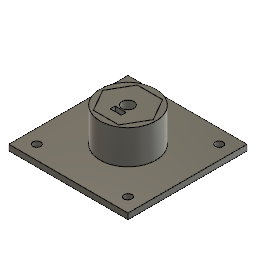
Rotation Motor Bottom Mount (Autodesk Fusion 360 design; units mm, degrees)
Autodesk Fusion 360 part; units mm, degrees
sketch "Sketch1" plane through (0, 0, 0) normal (0, 1, 0) x (1, 0, 0)
  circle A0 centre (-9.5106, -3.0902) radius 1.25
  circle A1 centre (0, 0) radius 14
  circle A2 centre (9.5106, -3.0902) radius 1.25
  circle A3 centre (5.8779, 8.0902) radius 1.25
  circle A4 centre (0, -10) radius 1.25
  circle A5 centre (5.8779, 8.0902) radius 1.25
  circle A6 centre (0, -10) radius 1.25
  circle A7 centre (-5.8779, 8.0902) radius 1.25
  circle A8 centre (9.5106, -3.0902) radius 1.25
  circle A9 centre (-9.5106, -3.0902) radius 1.25
  circle A10 centre (0, 0) radius 14
  circle A11 centre (-5.8779, 8.0902) radius 1.25
  circle A12 centre (-5.8779, 8.0902) radius 2.25
  circle A13 centre (5.8779, 8.0902) radius 2.25
  circle A14 centre (9.5106, -3.0902) radius 2.25
  circle A15 centre (0, -10) radius 2.25
  circle A16 centre (-9.5106, -3.0902) radius 2.25
  line L0 (30, -30) -> (-30, -30)
  line L1 (-30, -30) -> (-30, 30)
  line L2 (-30, 30) -> (30, 30)
  line L3 (30, 30) -> (30, -30)
  line L4 (30, -30) -> (-30, 30) construction
  line L5 (-30, -30) -> (30, 30) construction
  line L6 (-30, -30) -> (-22.9289, -22.9289)
  circle A17 centre (-22.9289, -22.9289) radius 1.95
  circle A18 centre (22.9289, -22.9289) radius 1.95
  circle A19 centre (22.9289, 22.9289) radius 1.95
  circle A20 centre (-22.9289, 22.9289) radius 1.95
  circle A21 centre (0, 0) radius 3
  line L7 (0, -3) -> (0, 2)
  line L8 (0, 2) -> (2.2361, 2)
  line L9 (0, 2) -> (-2.2361, 2)
  dimension "d13" = -1
  dimension "d14" = -1
  dimension "d15" = 1
  dimension "d16" = -1
  dimension "d17" = 1
  dimension "d33" = 60
  dimension "d34" = 60
  dimension "d35" = 10
  dimension "d36" = 3.9
  dimension "d50" = 6
  dimension "d51" = 5
  constraint horizontal L0
  constraint perpendicular L0 L1
  constraint parallel L0 L2
  constraint parallel L1 L3
  constraint parallel L5 L6
  constraint coincident L6.end A17.centre
  constraint coincident A1.centre A10.centre
  constraint coincident A21 L7.start
  constraint vertical L7
  constraint coincident A21 L8.end
  constraint perpendicular L7 L8
  constraint coincident A21 L9.end
  constraint perpendicular L7 L9
  measures "d33" distance of L1.end L2.end
  measures "d34" distance of L0.end L1.end
  measures "d35" distance of L0.end L6.end
  measures "d36" diameter of A17
  measures "d50" diameter of A21
  measures "d51" distance of L7.start L7.end
extrude "Extrude1" add sketch "Sketch1" along normal blind 17.065 contours A0 A9 | A1 A10 | A2 A8 | A3 A5 | A4 A6 | A7 A11 | A12 | A13 | A14 | A15 | A16 | A21 L7 L8 | A21 L8 L9 | A21 L7 L9 makes body 1
extrude "Extrude5" add sketch "Sketch1" 1 faces at (4.6394, 0, -2.5701) against normal blind 3 contours A0 A9 | A1 A10 | A2 A8 | A3 A5 | A4 A6 | A7 A11 | A12 | A13 | A14 | A15 | A16 | L0 L1 L2 L3 | A21 L7 L8 | A21 L8 L9 | A21 L7 L9 on bodies 1 bodies 1
sketch "Sketch3" plane through (0, 17.065, 0) normal (0, 1, 0) x (-1, 0, 0)
  circle A0 centre (0, 0) radius 14
  line L0 (6.3509, -11) -> (12.7017, 0)
  line L1 (12.7017, 0) -> (6.3509, 11)
  line L2 (6.3509, 11) -> (-6.3509, 11)
  line L3 (-6.3509, 11) -> (-12.7017, 0)
  line L4 (-12.7017, 0) -> (-6.3509, -11)
  line L5 (-6.3509, -11) -> (6.3509, -11)
  line L6 (-6.3797, 11.05) -> (-12.7594, 0)
  line L7 (-12.7594, 0) -> (-6.3797, -11.05)
  line L8 (-6.3797, -11.05) -> (6.3797, -11.05)
  line L9 (6.3797, -11.05) -> (12.7594, 0)
  line L10 (12.7594, 0) -> (6.3797, 11.05)
  line L11 (6.3797, 11.05) -> (-6.3797, 11.05)
  line L12 (0, -3) -> (0, 2)
  line L13 (0, 2) -> (2.2361, 2)
  circle A1 centre (0, 0) radius 3
  line L14 (0, 2) -> (-2.2361, 2)
  dimension "d55" = 11
  dimension "d56" = 0.05
  dimension "d61" = 6
  dimension "d62" = 5
  constraint coincident A0.centre A1.centre
  constraint coincident L12.start A1
  constraint vertical L12
  constraint coincident L13.end A1
  constraint perpendicular L12 L13
  constraint coincident L14.end A1
  constraint perpendicular L12 L14
  measures "d55" distance of A0.centre L5
  measures "d61" diameter of A1
  measures "d62" distance of L12.start L12.end
extrude "Extrude10" cut sketch "Sketch3" against normal blind 17.065 contours L0 L1 L2 L3 L4 L5 | L6 L7 L8 L9 L10 L11 | L12 A1 L14 | L12 L13 A1 | L13 A1 L14 bodies 1
extrude "Extrude11" add sketch "Sketch3" against normal blind 15 separate body contours L0 L1 L2 L3 L4 L5 | L12 A1 L14 | L12 L13 A1 | L13 A1 L14 makes body 2
extrude "Extrude12" cut sketch "Sketch3" against normal up to surface (15 mm away) contours L12 A1 L14 | L12 L13 A1 bodies 2
extrude "Extrude13" cut sketch "Sketch3" against normal blind 2 contours L13 A1 L14 bodies 2
sketch "Sketch4" plane through (0, 0, 11) normal (0, 0, 1) x (1, 0, 0)
  line L0 (6.3509, 17.065) -> (-6.3509, 17.065)
  line L1 (-6.3509, 17.065) -> (-6.3509, 2.065)
  line L2 (-6.3509, 2.065) -> (6.3509, 2.065)
  line L3 (6.3509, 2.065) -> (6.3509, 17.065)
  line L4 (0, 2.065) -> (0, 17.065)
  circle A0 centre (0, 9.565) radius 1.5
  circle A1 centre (0, 9.565) radius 2.75
  line L5 (-2.75, 7.9773) -> (0, 6.3896)
  line L6 (0, 6.3896) -> (2.75, 7.9773)
  line L7 (2.75, 7.9773) -> (2.75, 11.1527)
  line L8 (2.75, 11.1527) -> (0, 12.7404)
  line L9 (0, 12.7404) -> (-2.75, 11.1527)
  line L10 (-2.75, 11.1527) -> (-2.75, 7.9773)
  line L11 (-2.75, 11.1527) -> (-2.75, 17.065)
  line L12 (2.75, 11.1527) -> (2.75, 17.065)
  point P0 (0, 9.565)
  dimension "d67" = 3
  dimension "d68" = 5.5
  dimension "d73" = 2.75
  constraint midpoint L2 L4.start
  constraint midpoint L0 L4.end
  constraint midpoint L4 P0
  constraint concentric A0 A1
  constraint coincident P0 A0.centre
  constraint coincident L0 L11.end
  constraint perpendicular L0 L11
  constraint coincident L0 L12.end
  constraint perpendicular L0 L12
  measures "d67" diameter of A0
  measures "d68" diameter of A1
  measures "d73" distance of P0 L10
extrude "Extrude14" cut sketch "Sketch4" against normal blind 3.2 contours L4 A0 A1 | L4 A0 A1 bodies 2
extrude "Extrude15" cut 1 faces at (0.9997, 9.2227, 11) along direction (0, 0, -1) up to surface (9 mm away) on bodies 2 bodies 2
extrude "Extrude16" cut sketch "Sketch4" along normal blind 2.4 from surface at -7.3 contours L0 L4 L8 L12 | L0 L4 L9 L11 | A1 L7 L8 | L4 A1 L8 | L4 A1 L9 | L4 A0 A1 | A1 L6 L7 | L4 A1 L5 | L4 A1 L6 | A1 L9 L10 | L4 A0 A1 | A1 L5 L10 | L4 A0 | L4 A0 bodies 2
extrude "Extrude8" [suppressed]
extrude "Extrude9" [suppressed]
extrude "Extrude7" [suppressed]
equation "d1 = 7.065 mm + 10 mm"
equation "d43 = 20.065 mm - 15 mm"
equation "d59 = -17.065 mm + 2.065 mm"
equation "d73 = 5.5 mm / 2"
equation "d76 = -3.2 mm + ( -5.8 / 2 ) * 1 mm + ( -2.4 / 2 ) * 1 mm"
